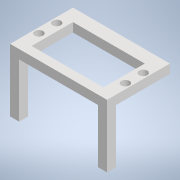
# Autodesk Inventor part: держатель_сервы
Saved by Autodesk Inventor 2021.1 (Build 251245010, 245A)
## iProperties
Created: 2022-12-17
Part Number: держатель_сервы
Material: Типовые
Document SubType Name: Modeling
Designer: zmoze
Density: 1 g/cm^3
Appearance: По умолчанию
Author: zmoze
Autodesk Inventor part; units mm, degrees
ref_plane "YZ Plane" through (0, 0, 0) normal (1, 0, 0) x (0, 1, 0)
ref_plane "XZ Plane" through (0, 0, 0) normal (0, 1, 0) x (-1, 0, 0)
ref_plane "XY Plane" through (0, 0, 0) normal (0, 0, 1) x (1, 0, 0)
sketch "Эскиз1" plane through (0, 0, 0) normal (0, 0, 1) x (1, 0, 0)
  line L0 (-27, 0) -> (27, 0)
  line L1 (27, 0) -> (27, -5)
  line L2 (27, -5) -> (-27, -5)
  line L3 (-27, -5) -> (-27, 0)
  line L4 (27, -5) -> (22, -5)
  line L5 (22, -5) -> (22, -35)
  line L6 (22, -35) -> (27, -35)
  line L7 (27, -35) -> (27, -5)
  line L8 (-27, -5) -> (-22, -5)
  line L9 (-22, -5) -> (-22, -35)
  line L10 (-22, -35) -> (-27, -35)
  line L11 (-27, -35) -> (-27, -5)
  point P0 (0, 0)
  point P1 (0, 0)
  point P2 (-22, -5)
  point P3 (22, -5)
  dimension "d0" = 35
  dimension "d1" = 5
  dimension "d2" = 54
  dimension "d3" = 5
  constraints: 24 end point, 6 parallel, 3 horizontal, 3 perpendicular, 1 coincident, 1 collinear, 1 midpoint, 1 point on line
  measures "d0" distance of L10.end L0.start
  measures "d1" distance of L2.end L0.start
  measures "d2" distance of L0.start L0.end
  measures "d3" distance between parallel lines of L5 L7
extrude "Выдавливание1" add sketch "Эскиз1" along normal blind 5
sketch "Эскиз3" plane through (-27, 0, 0) normal (0, 1, 0) x (1, 0, 0)
  line L0 (0, 0) -> (7, 0)
  line L1 (7, 0) -> (7, 23)
  line L2 (7, 23) -> (0, 23)
  line L3 (0, 23) -> (0, 0)
  line L4 (0, 23) -> (54, 23)
  line L5 (54, 23) -> (54, 30)
  line L6 (54, 30) -> (0, 30)
  line L7 (0, 30) -> (0, 23)
  line L8 (54, 0) -> (0, 0) projected
  line L9 (54, 23) -> (47, 23)
  line L10 (47, 23) -> (47, 0)
  line L11 (47, 0) -> (54, 0)
  line L12 (54, 0) -> (54, 23)
  line L13 (54, 0) -> (54, -5) projected
  point P0 (27, 0)
  point P1 (54, 0)
  dimension "d6" = 7
  dimension "d7" = 7
  dimension "d8" = 7
  dimension "d9" = 23
  constraints: 24 end point, 6 parallel, 3 horizontal, 3 perpendicular, 1 collinear, 1 point on line
  measures "d6" distance between parallel lines of L12 L10
  measures "d7" distance between parallel lines of L3 L1
  measures "d8" distance between parallel lines of L4 L6
  measures "d9" distance between parallel lines of L8 L4
extrude "Выдавливание2" add sketch "Эскиз3" against normal blind 5 contours L3 L2 L1 L0 | L7 L6 L5 L4 L2 | L10 L4 L12 L8
sketch "Эскиз4" plane through (-27, 0, 5) normal (0, 1, 0) x (1, 0, 0)
  arc A0 (52.8363, 24.448) -> (52.8363, 21.648) centre (51.075, 23.048) ccw projected
  arc A1 (52.8363, 14.542) -> (52.8363, 11.742) centre (51.075, 13.142) ccw projected
  arc A2 (1.1636, 11.742) -> (1.1636, 14.542) centre (2.925, 13.142) ccw projected
  arc A3 (1.1636, 21.648) -> (1.1636, 24.448) centre (2.925, 23.048) ccw projected
  circle A4 centre (51.075, 23.048) radius 2.25
  circle A5 centre (51.075, 13.142) radius 2.25
  circle A6 centre (2.925, 13.142) radius 2.25
  circle A7 centre (2.925, 23.048) radius 2.25
  point P0 (27, 5)
  point P1 (1.1636, 24.448)
  point P2 (1.1636, 14.542)
  point P3 (52.8363, 11.742)
  point P4 (52.8363, 24.448)
  constraints: 4 coincident, 12 other
extrude "Выдавливание3" cut sketch "Эскиз4" against normal blind 5
